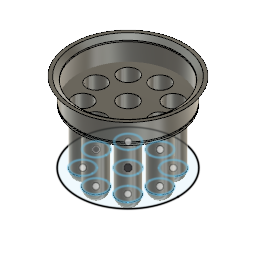
enz one part 0 v1 (Autodesk Fusion 360 design; units mm, degrees)
Autodesk Fusion 360 part; units mm, degrees
sketch "base" plane through (0, 0, 0) normal (0, 0, 1) x (1, 0, 0)
  circle A0 centre (-21, 0.0874) radius 6.2
  circle A1 centre (-21, 0.0874) radius 6.8
  circle A2 centre (0, 0) radius 32.9
  circle A3 centre (0, 0) radius 6.8
  circle A4 centre (-14.911, -14.7874) radius 6.8
  circle A5 centre (-0.0874, -21) radius 6.8
  circle A6 centre (14.7874, -14.911) radius 6.8
  circle A7 centre (21, -0.0874) radius 6.8
  circle A8 centre (14.911, 14.7874) radius 6.8
  circle A9 centre (0.0874, 21) radius 6.8
  circle A10 centre (-14.7874, 14.911) radius 6.8
  circle A11 centre (-14.911, -14.7874) radius 6.2
  circle A12 centre (-0.0874, -21) radius 6.2
  circle A13 centre (14.7874, -14.911) radius 6.2
  circle A14 centre (21, -0.0874) radius 6.2
  circle A15 centre (14.911, 14.7874) radius 6.2
  circle A16 centre (0.0874, 21) radius 6.2
  circle A17 centre (-14.7874, 14.911) radius 6.2
  circle A18 centre (0, 0) radius 6.2
  point P0 (-21, 0.0874)
  dimension "d6" = 13.6
  dimension "d54" = 13.6
  dimension "d65" = 360
  dimension "d67" = 21
  dimension "d68" = 12.4
  dimension "d84" = 65.8
  dimension "d146" = 12.4
  constraint concentric A0 A1
  constraint coincident A2.centre A3.centre
  constraint coincident P0 A0.centre
  constraint concentric A3 A18
  measures "d6" diameter of A1
  measures "d54" diameter of A3
  measures "d67" horizontal distance of P0 A2.centre
  measures "d68" diameter of A0
  measures "d84" diameter of A2
  measures "d146" diameter of A18
sketch "domeBottom" plane through (0, 0, 0) normal (0, 1, 0) x (1, 0, 0)
  arc A0 (-20.9888, 6.2) -> (-27.1888, 0) centre (-20.9888, 0) ccw
  arc A1 (-20.9888, 6.8) -> (-27.7888, 0) centre (-20.9888, 0) ccw
  arc A2 (-20.9888, 6.2) -> (-27.1888, 0) centre (-20.9888, 0) ccw
  line L0 (-27.7888, 0) -> (-27.1888, 0)
  line L1 (-14.7888, 0.0103) -> (-14.1888, 0.0103)
  line L2 (-20.9888, 0) -> (-20.9888, 6.8) construction
  line L3 (-20.9888, 6.2) -> (-20.9888, 6.8)
  line L4 (-6.8, -0.0034) -> (6.8, -0.0034)
  arc A3 (0, 6.8) -> (-6.8, -0.0034) centre (0, 0) ccw
  arc A4 (0, 6.2) -> (-6.2, -0.0034) centre (0, 0) ccw
  line L5 (0, 0) -> (0, 6.8)
  dimension "d110" = 6.8
  dimension "d111" = 6.2
  dimension "d152" = 6.8
  dimension "d153" = 6.2
  constraint concentric A0 A2
  constraint concentric A0 A1
  constraint horizontal L0
  constraint parallel L0 L1
  constraint coincident A0.centre A1.centre
  constraint vertical L2
  constraint coincident L2 A0.start
  constraint coincident A0.centre L0
  constraint coincident A3.centre A4.centre
  constraint horizontal L4
  constraint coincident L4 A4.end
  constraint perpendicular L4 L5
  constraint coincident L5 A4.start
  measures "d110" radius of A1
  measures "d111" radius of A0
  measures "d152" radius of A3
  measures "d153" radius of A4
extrude "sideTube" add sketch "base" along normal blind 38 contours A1 makes body 1
extrude "Extrude16" add sketch "base" along normal blind 38 separate body contours A3 makes body 2
revolve "Revolve3" add sketch "domeBottom" angle 360 about axis through (-20.9888, 0, 0) along (0, 0, -1) contours A0 A1 A2 L0 L3 bodies 1
revolve "Revolve4" add sketch "domeBottom" angle 360 about axis through (0, 0, 1.75) along (0, 0, 1) contours L4 A3 A4 L5 bodies 2
pattern_circular "C-Pattern1" count 8 over 360 about axis through (0, 0, 1.75) along (0, 0, 1) of bodies 1 makes body 3 at (-10.8701, -20.2565, 25.3333) makes body 4 at (6.6372, -22.0098, 25.3333) makes body 5 at (20.2565, -10.8701, 25.3333) makes body 6 at (22.0098, 6.6372, 25.3333) makes body 7 at (10.8701, 20.2565, 25.3333) makes body 8 at (-6.6372, 22.0098, 25.3333) makes body 9 at (-20.2565, 10.8701, 25.3333)
extrude "Extrude17" add sketch "base" along normal blind 2 from surface at 36 contours A2 bodies 1 3 4 5 6 7 8 9 2
fillet "Fillet19" radius 1 9 edges at (-2.5464, -27.3398, 36) (-21.1327, -17.5316, 36) (-27.3398, 2.5464, 36) (-17.5316, 21.1327, 36) (17.5316, -21.1327, 36) (27.3398, -2.5464, 36) (21.1327, 17.5316, 36) (2.5464, 27.3398, 36) (-6.3398, 2.459, 36) on bodies 1
sketch "rim" plane through (0, 0, 0) normal (0, 1, 0) x (1, 0, 0)
  line L0 (32.9, -37.2) -> (32.9, -49.2)
  line L1 (31.9, -49.196) -> (32.9, -49.2)
  line L2 (32.9, -49.2) -> (37.25, -52.1593)
  line L3 (31.8966, -50.0514) -> (34.9952, -52.1593)
  line L4 (34.9952, -52.1593) -> (37.25, -52.1593)
  line L5 (31.9, -49.196) -> (32.9, -49.2)
  line L6 (31.9, -49.196) -> (31.9, -37.2)
  line L7 (31.9, -49.196) -> (31.8966, -50.0514)
  line L8 (32.9, -37.2) -> (31.9, -37.2)
  point P0 (32.9, -37.2)
  dimension "d26" = 37.2
  dimension "d27" = 32.9
  dimension "d29" = 12
  dimension "d63" = 37.25
  dimension "d75" = 34
  dimension "d101" = 31.9
  dimension "d103" = 1
  constraint coincident P0 L0.start
  constraint parallel L2 L3
  constraint horizontal L4
  constraint perpendicular L1 L7
  constraint perpendicular L6 L8
  constraint parallel L0 L6
  measures "d26" vertical distance of origin L0.start
  measures "d27" horizontal distance of P0 origin
  measures "d29" distance of P0 L0.end
  measures "d63" horizontal distance of L2.end origin
  measures "d75" angle of L2 L5
  measures "d101" horizontal distance of origin L1.start
  measures "d103" horizontal distance of L6.end P0
revolve "Revolve2" add sketch "rim" angle 360 about axis through (0, 0, 1.75) along (0, 0, 1) separate body makes body 10
sketch "washerMold" plane through (0, 0, 0) normal (0, 0, 1) x (1, 0, 0)
  circle A0 centre (0, 0) radius 37.25
  circle A1 centre (0, 0) radius 32.9
  circle A2 centre (0, 0) radius 32.15
  circle A3 centre (0, 0) radius 38
  dimension "d85" = 74.5
  dimension "d86" = 65.8
  dimension "d87" = 76
  dimension "d88" = 64.3
  constraint concentric A0 A1
  constraint concentric A0 A2
  constraint concentric A2 A3
  measures "d85" diameter of A0
  measures "d86" diameter of A1
  measures "d87" diameter of A3
  measures "d88" diameter of A2
extrude "Extrude12" add sketch "washerMold" along normal blind 5 separate body makes body 11 at (37.8112, -3.7836, 1.6667) makes body 12 at (32.8591, -1.6399, 3.3333)
extrude "Extrude13" add sketch "washerMold" along normal blind 2 contours A0 bodies 11 12
chamfer "Chamfer1" distance 0.3 angle 45 1 edges at (-30.6736, -11.8971, 2) on bodies 11
chamfer "Chamfer2" distance 0.3 angle 45 1 edges at (-34.7292, 13.4702, 2) on bodies 11
hidden bodies 11
equation "d6 = tubeInsideDiameter + DoubleTubeWallThickness"
equation "submergedTubeHeight = 36 mm"
equation "capHeightAndOverhead = 12 mm"
equation "tubeInsideDiameter = 12.4 mm"
equation "largeRimOutsideDiameter = 74.5 mm"
equation "baseRimOutsideDiameter = 65.8 mm"
equation "generalThickness = 2 mm"
equation "DoubleTubeWallThickness = 1.2 mm"
equation "d26 = submergedTubeHeight + DoubleTubeWallThickness"
equation "d27 = baseRimOutsideDiameter / 2"
equation "d29 = capHeightAndOverhead"
equation "d39 = submergedTubeHeight + tubeBottomThickness"
equation "d54 = tubeInsideDiameter + DoubleTubeWallThickness"
equation "d63 = largeRimOutsideDiameter / 2"
equation "d65 = 360.00 °"
equation "tubeBottomThickness = 2 mm"
equation "d67 = outsideTubeToCenterTube"
equation "d68 = tubeInsideDiameter"
equation "d75 = 34 °"
equation "d84 = baseRimOutsideDiameter"
equation "d85 = largeRimOutsideDiameter"
equation "d86 = baseRimOutsideDiameter"
equation "d87 = largeRimOutsideDiameter + 1.5 mm"
equation "d88 = baseRimOutsideDiameter - 1.5 mm"
equation "d101 = baseRimOutsideDiameter / 2 - reolvedPartThickness"
equation "reolvedPartThickness = 1 mm"
equation "d103 = reolvedPartThickness"
equation "d110 = ( tubeInsideDiameter + DoubleTubeWallThickness ) / 2"
equation "d111 = tubeInsideDiameter / 2"
equation "outsideTubeToCenterTube = 21 mm"
equation "d146 = tubeInsideDiameter"
equation "d152 = ( tubeInsideDiameter + DoubleTubeWallThickness ) / 2"
equation "d153 = tubeInsideDiameter / 2"
equation "d156 = submergedTubeHeight + tubeBottomThickness"
equation "d159 = submergedTubeHeight"
equation "d160 = tubeBottomThickness"
named bodies: "holderRim", "washer mold", "domeBottom (1)", "domeBottom (2)", "domeBottom (3)", "domeBottom (4)", "domeBottom (5)", "domeBottom (6)", "domeBottom (7)", "centerTube", "sideTube"
